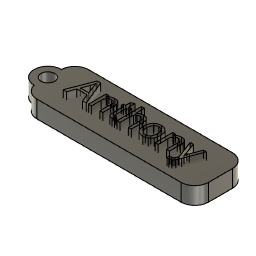
Excerise 1 v1 (Autodesk Fusion 360 design; units mm, degrees)
Autodesk Fusion 360 part; units mm, degrees
sketch "Sketch1" plane through (0, 0, 0) normal (0, 0, 1) x (1, 0, 0)
  line L0 (4.0006, 7.8958) -> (46, 7.8958)
  line L1 (50, 3.8958) -> (50, -3.1042)
  line L2 (46, -7.1042) -> (4.0073, -7.1042)
  circle A0 centre (0, 0) radius 4
  circle A1 centre (0, 0) radius 2
  arc A2 (46, -7.1042) -> (50, -3.1042) centre (46, -3.1042) ccw
  arc A3 (50, 3.8958) -> (46, 7.8958) centre (46, 3.8958) ccw
  line L3 (4.0006, 7.8958) -> (4.0006, 7.8958)
  line L4 (3.8976, -7.1042) -> (4.0073, -7.1042)
  arc A4 (4.0006, 7.8958) -> (0.0015, 4) centre (4.0001, 3.8958) ccw
  arc A5 (-0.0008, -4) -> (3.8976, -7.1042) centre (3.8976, -3.1042) ccw
  line L5 (-0.0008, -4) -> (0.0015, 4) construction
  line L6 (7.3567, -5) -> (44.4351, -5) construction
  line L7 (44.4351, -5) -> (44.4351, 5) construction
  line L8 (44.4351, 5) -> (7.3567, 5) construction
  line L9 (7.3567, 5) -> (7.3567, -5) construction
  line L10 (0, 0) -> (7.3567, 0) construction
  line L11 (7.3567, 5) -> (7.3567, 7.8958) construction
  point P0 (0, 7.8958)
  point P1 (50, 7.8958)
  point P2 (0.0073, -7.1042)
  dimension "d1" = 50
  dimension "d2" = 15
  dimension "d3" = 8
  dimension "d4" = 4
  dimension "d7" = 4
  dimension "d8" = 4
  dimension "d9" = 4
  dimension "d10" = 4
  text T0 "Anthony" font "Arial" height 10 align ink ink in box 0 x 0 at (7.3567, -5) x (1, 0) y (0, 1) spacing 1 height is em
  constraint horizontal L0
  constraint vertical L1
  constraint horizontal L2
  constraint coincident A0.centre A1.centre
  constraint coincident P0 L0
  constraint coincident P2 L2
  constraint tangent L1 A2
  constraint tangent L2 A2
  constraint coincident P1 L0
  constraint coincident P1 L1
  constraint tangent L0 A3
  constraint tangent L1 A3
  constraint parallel L2 L4
  constraint tangent L4 A5
  constraint coincident A0 A5.start
  constraint coincident A0 A4.end
  constraint perpendicular L6 L7
  constraint parallel L6 L8
  constraint parallel L7 L9
  constraint perpendicular L9 L10
  constraint midpoint L9 L10.end
  constraint parallel L2 L10
  constraint coincident L0 L11.end
  constraint perpendicular L0 L11
  measures "d1" distance of P0 P1
  measures "d2" distance of P0 P2
  measures "d3" diameter of A0
  measures "d4" diameter of A1
  measures "d7" radius of A2
  measures "d8" radius of A3
  measures "d9" radius of A4
  measures "d10" radius of A5
extrude "Extrude2" add sketch "Sketch1" along normal blind 7 text T0 makes body 1 at (14.7105, -1.147, 2.3333) makes body 2 at (43.3303, 0.5522, 2.3333) makes body 3 at (28.3099, 0.1517, 3.5) makes body 4 at (34.1734, -1.147, 2.3333) makes body 5 at (23.0503, 1.8966, 4.6667) makes body 6 at (21.3072, 0.6157, 2.3333) makes body 7 at (13.0894, -0.4894, 2.3333)
extrude "Extrude1" add sketch "Sketch1" along normal blind 5 separate body makes body 8
